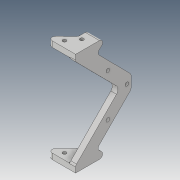
# Autodesk Inventor part: frameBracket
Saved by Autodesk Inventor 2018 (Build 220112000, 112)
## iProperties
Created: 2020-03-12
Part Number: frameBracket
Material: Generic
Document SubType Name: Modeling
Designer: anirudh
Density: 1 g/cm^3
Appearance: Default
Author: anirudh
Autodesk Inventor part; units mm, degrees
ref_plane "YZ Plane" through (0, 0, 0) normal (1, 0, 0) x (0, 1, 0)
ref_plane "XZ Plane" through (0, 0, 0) normal (0, 1, 0) x (-1, 0, 0)
ref_plane "XY Plane" through (0, 0, 0) normal (0, 0, 1) x (1, 0, 0)
sketch "Sketch3" plane through (0, 0, 0) normal (1, 0, 0) x (0, 1, 0)
  line L0 (40.6077, -164.606) -> (27.4372, -164.606)
  arc A0 (30.4525, -150.234) -> (37.5924, -150.234) centre (34.0225, -146.6199) ccw
  arc A1 (30.4525, -150.234) -> (37.5924, -150.234) centre (34.0225, -146.6199) ccw
  circle A2 centre (34.0225, -160.4375) radius 1.8
  circle A3 centre (34.0225, -160.4375) radius 1.8
  circle A4 centre (55.0753, -141.6399) radius 1.8
  circle A5 centre (55.0753, -141.6399) radius 1.8
  circle A6 centre (12.9696, -141.6399) radius 1.8
  circle A7 centre (12.9696, -141.6399) radius 1.8
  line L1 (-9.1845, -133.2731) -> (-16.7775, -141.5399)
  arc A8 (-9.5, -110.7696) -> (-11.7313, -109.8534) centre (-11.7313, -113.0284) ccw
  arc A9 (-9.5, -110.7696) -> (-11.7313, -109.8534) centre (-11.7313, -113.0284) ccw
  line L2 (-16.7775, -109.8534) -> (-16.7775, -141.5399)
  line L3 (-16.7775, -109.8534) -> (-16.7775, -141.5399)
  line L4 (-11.7313, -109.8534) -> (-16.7775, -109.8534)
  line L5 (-11.7313, -109.8534) -> (-16.7775, -109.8534)
  arc A10 (-4.5133, -133.0459) -> (-9.1845, -133.2731) centre (-6.7445, -135.3047) ccw
  arc A11 (79.7762, -109.8534) -> (77.5449, -110.7696) centre (79.7762, -113.0284) ccw
  arc A12 (79.7762, -109.8534) -> (77.5449, -110.7696) centre (79.7762, -113.0284) ccw
  line L6 (84.8225, -109.8534) -> (79.7762, -109.8534)
  line L7 (79.7762, -109.8534) -> (84.8225, -109.8534)
  arc A13 (77.2294, -133.2731) -> (72.5582, -133.0459) centre (74.7895, -135.3047) ccw
  line L8 (84.8225, -109.8534) -> (84.8225, -141.5399)
  line L9 (84.8225, -141.5399) -> (77.2294, -133.2731)
  line L10 (72.5582, -133.0459) -> (40.6077, -164.606)
  line L11 (27.4372, -164.606) -> (-4.5133, -133.0459)
  line L12 (77.5449, -110.7696) -> (37.5924, -150.234)
  line L13 (30.4525, -150.234) -> (-9.5, -110.7696)
  point P0 (-9.9195, -135.3047)
  constraints: 26 end point, 17 point on circle, 14 centre point, 8 coincident, 7 tangent, 2 collinear, 2 parallel, 1 vertical, 3 other
extrude "Extrusion2" add sketch "Sketch3" along normal blind 5.588
sketch "Sketch4" plane through (0, 84.8225, -109.8534) normal (0, 1, 0) x (1, 0, 0)
  arc A0 (130.2317, 79.7227) -> (128.1154, 80.5308) centre (128.1154, 77.3558) ccw
  arc A1 (130.2317, 79.7227) -> (128.1154, 80.5308) centre (128.1154, 77.3558) ccw
  line L0 (114.4229, 88.9128) -> (114.4229, 80.5308)
  circle A2 centre (122.3477, 84.7218) radius 1.75
  circle A3 centre (139.9473, 77.3558) radius 1.75
  line L1 (146.1221, 63.5783) -> (130.2317, 79.7227)
  line L2 (128.1154, 80.5308) -> (114.4229, 80.5308)
  line L3 (114.4229, 88.9128) -> (146.1221, 88.9128)
  line L4 (146.1221, 88.9128) -> (146.1221, 63.5783)
  line L5 (0, 0) -> (5.588, 0) projected
  line L6 (0, 0) -> (-25.3238, 0)
  line L7 (0, 31.6865) -> (5.588, 31.6865) projected
  line L8 (0, 0) -> (0, 31.6865)
  line L9 (0, 31.6865) -> (-8.382, 31.6865)
  line L10 (-8.382, 31.6865) -> (-8.382, 17.9959)
  line L11 (-25.3238, 0) -> (-9.1777, 15.8945)
  line L12 (-25.3238, 0) -> (-2.667, 0) construction
  arc A4 (-9.1777, 15.8945) -> (-8.382, 17.9959) centre (-11.557, 17.9967) ccw
  line L13 (-4.191, 31.6865) -> (-4.191, 0)
  line L14 (-4.191, 15.8432) -> (-4.191, 31.6865)
  circle A5 centre (-11.557, 6.1722) radius 1.75
  circle A6 centre (-4.191, 15.8432) radius 1.75
  point P0 (0, -109.8534)
  dimension "d19" = 3.5
  constraints: 26 end point, 7 centre point, 6 point on circle, 5 horizontal, 3 perpendicular, 2 coincident, 2 midpoint, 2 tangent, 2 vertical, 1 collinear, 1 equal length, 1 point on line
  measures "d19" diameter of A6
extrude "Extrusion5" add sketch "Sketch4" against normal blind 5.588 contours L6 L13 A6 L9 L8 | L6 L11 A4 L10 L9 L13 A6
sketch "Sketch6" plane through (0, 79.2345, -141.5399) normal (1, 0, 0) x (0, 0, -1)
  line L0 (-6.0838, 0) -> (0, 5.588) projected
  line L1 (0, 0) -> (-6.0838, 0) projected
  line L2 (0, 5.588) -> (0, 0)
  line L3 (0, 0) -> (-6.0838, 0)
  line L4 (0, 5.588) -> (-31.6865, 5.588) projected
  line L5 (-6.0838, 0) -> (0, 5.588)
  point P0 (-141.5399, -79.2345)
  constraints: 6 end point, 2 perpendicular
extrude "Extrusion6" cut sketch "Sketch6" against normal blind 27.7495
ref_plane "Work Plane1" through (5.588, 34.0225, -109.8534) normal (0, 1, 0) x (1, 0, 0)
mirror "Mirror1" about plane through (5.588, 34.0225, -109.8534) normal (0, 1, 0) of "Extrusion5", "Extrusion6"
fillet "Fillet1" radius 3.175 2 edges at (-25.3238, 82.0285, -109.8534) (-25.3238, -13.9835, -109.8534)
fillet "Fillet2" radius 3.175 2 edges at (-1.397, 84.8225, -141.5399) (-1.397, -16.7775, -141.5399)
fillet "Fillet3" radius 3.175 2 edges at (2.794, 40.6077, -164.606) (2.794, 27.4372, -164.606)
fillet "Fillet4" radius 1.27 2 edges at (0, 79.2345, -122.678) (0, -11.1895, -122.678)
body "Solid2"
